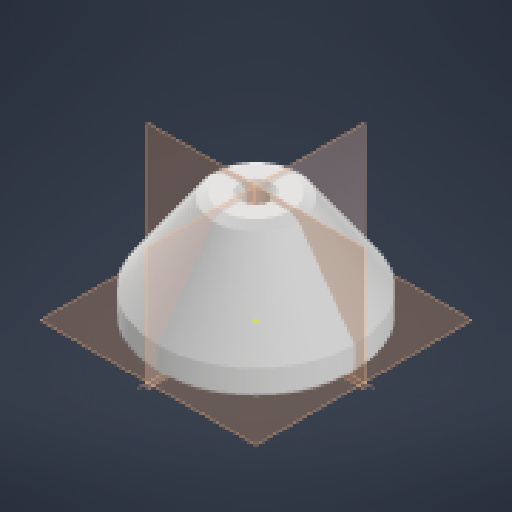
# Autodesk Inventor part: PesaGrua
Saved by Autodesk Inventor 2026.2 (Build 302298010, 298A)
## iProperties
Created: 2026-04-23
Part Number: PesaGrua
Material: Genérico
Document SubType Name: Modeling
Designer: Jose Carlos
Density: 1 g/cm^3
Appearance: Valor por defecto
Author: Jose Carlos
Autodesk Inventor part; units mm, degrees
sketch "Boceto1" plane through (0, 0, 0) normal (0, 1, 0) x (-1, 0, 0)
  line L0 (-12.5, -12.5) -> (12.5, -12.5) construction
  line L1 (12.5, -12.5) -> (12.5, 12.5) construction
  line L2 (12.5, 12.5) -> (-12.5, 12.5) construction
  line L3 (-12.5, 12.5) -> (-12.5, -12.5) construction
  line L4 (-12.5, -12.5) -> (12.5, 12.5) construction
  line L5 (12.5, -12.5) -> (-12.5, 12.5) construction
  circle A0 centre (0, 0) radius 17.6777
  dimension "d0" = 25
  dimension "d1" = 25
  constraints: 12 end point, 2 midpoint, 2 parallel, 1 coincident, 1 horizontal, 1 perpendicular, 3 other
  measures "d0" distance of L0.end L1.end
  measures "d1" distance of L1.end L2.end
extrude "Extrusión1" add sketch "Boceto1" along normal blind 5
sketch "Boceto2" plane through (0, 0, 0) normal (1, 0, 0) x (0, 1, 0)
  line L0 (5, -17.6777) -> (5, 17.6777) construction
  line L1 (5, 0) -> (30, 0)
  line L2 (30, 0) -> (5, 17.6777)
  line L3 (20, 0) -> (20, 7.0711)
  line L4 (5, 0) -> (5, 17.6777)
  line L5 (-6, 0) -> (36, 0) projected
  point P0 (0, 0)
  dimension "d4" = 25
  dimension "d5" = 15
  constraints: 8 end point, 2 point on line, 1 horizontal, 1 midpoint, 1 perpendicular
  measures "d4" distance of L1.start L1.end
  measures "d5" distance between parallel lines of L0 L3
revolve "Revolución1" add sketch "Boceto2" angle 360 about axis through (0, -10, 0) along (0, 1, 0) contours L4 L2 L3 L1
sketch "Boceto3" plane through (0, 20, 0) normal (0, 1, 0) x (1, 0, 0)
  point P0 (0, 0)
  point P1 (0, 0)
  constraints: 1 coincident
hole "Agujero1" at (0, 20, 0) direction (0, -1, 0) diameter 3.6 end through all
sketch "Boceto4" plane through (0, 0, 0) normal (0, -1, 0) x (1, 0, 0)
  point P0 (0, 0)
chamfer "Chaflán1" distance 4 angle 45 1 edges at (0, 0, -1.8)
chamfer "Chaflán2" distance 1 angle 45 2 edges at (17.6777, 0, 0) (0, 20, -7.0711)
chamfer "Chaflán3" distance 1 angle 45 1 edges at (0, 20, -1.8)
